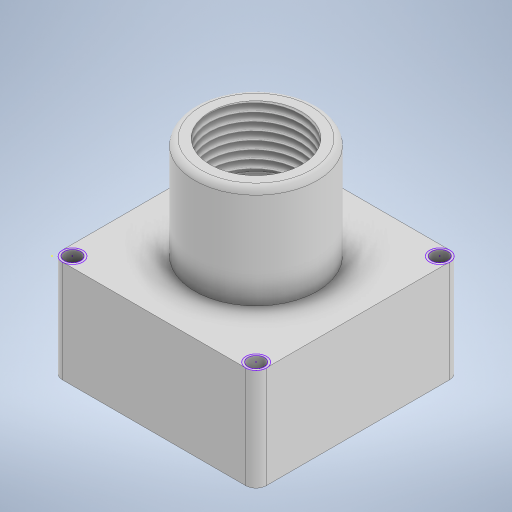
# Autodesk Inventor part: Practica1 - Jonnathan Lanuza
Saved by Autodesk Inventor 2024 (Build 280153000, 153)
## iProperties
Created: 2024-02-19
Part Number: Practica1 - Jonnathan Lanuza
Material: Generic
Document SubType Name: Modeling
Designer: Jonnathan Lanuza
Density: 1 g/cm^3
Appearance: Default
Author: Jonnathan Lanuza
Title: Practica 1 - Dinamica
Autodesk Inventor part; units mm, degrees
ref_plane "YZ Plane" through (0, 0, 0) normal (1, 0, 0) x (0, 1, 0)
ref_plane "XZ Plane" through (0, 0, 0) normal (0, 1, 0) x (-1, 0, 0)
ref_plane "XY Plane" through (0, 0, 0) normal (0, 0, 1) x (1, 0, 0)
sketch "Sketch1" plane through (0, 0, 0) normal (0, 1, 0) x (-1, 0, 0)
  point P0 (0, 0)
sketch "Sketch2" plane through (0, 0, 0) normal (0, 1, 0) x (-1, 0, 0)
  line L0 (-50, 50) -> (50, 50)
  line L1 (50, 50) -> (50, -50)
  line L2 (50, -50) -> (-50, -50)
  line L3 (-50, -50) -> (-50, 50)
  line L4 (-50, 50) -> (50, -50) construction
  line L5 (50, 50) -> (-50, -50) construction
  point P0 (0, 0)
  dimension "d0" = 100
  dimension "d1" = 100
  constraints: 12 end point, 2 midpoint, 2 parallel, 1 horizontal, 1 perpendicular
  measures "d0" distance of L1.end L2.end
  measures "d1" distance of L0.end L1.end
extrude "Extrusion1" add sketch "Sketch2" against normal blind 50
sketch "Sketch3" plane through (0, 0, 0) normal (0, 1, 0) x (1, 0, 0)
  circle A0 centre (0, 0) radius 30
  dimension "d4" = 60
  constraints: 1 centre point, 1 coincident
  measures "d4" diameter of A0
extrude "Extrusion2" add sketch "Sketch3" along normal blind 50
sketch "Sketch4" plane through (0, 50, 0) normal (0, 1, 0) x (1, 0, 0)
  point P0 (0, 0)
hole "Hole1" at (0, 50, 0) direction (0, -1, 0) diameter 45 depth 30
thread "Thread1" size "M50x4" class "6H" standard "ANSI Metric M Profile" full length
fillet "Fillet1" radius 3 1 edges at (-30, 50, 0)
sketch "Sketch9" plane through (0, 0, 0) normal (0, 1, 0) x (1, 0, 0)
  circle A0 centre (45, 45) radius 4
  circle A1 centre (45, 45) radius 5
  circle A2 centre (45, -45) radius 5
  circle A3 centre (45, -45) radius 4
  circle A4 centre (-45, 45) radius 4
  circle A5 centre (-45, 45) radius 5
  circle A6 centre (-45, -45) radius 4
  circle A7 centre (-45, -45) radius 5
  point P0 (0, 0)
  point P1 (-50, 50)
  point P2 (-50, -50)
  constraints: 8 centre point, 4 coincident
fillet "Fillet6" radius 5 1 edges at (-50, -25, 50)
fillet "Fillet7" radius 5 1 edges at (-50, -25, -50)
fillet "Fillet8" radius 5 1 edges at (50, -25, -50)
fillet "Fillet9" radius 5 1 edges at (50, -25, 50)
hole "Hole7" at (45, 0, -45) direction (0, -1, 0) diameter 8 end through all
hole "Hole8" at (45, 0, 45) direction (0, -1, 0) diameter 8 end through all
hole "Hole9" at (-45, 0, 45) direction (0, -1, 0) diameter 8 end through all
hole "Hole10" at (-45, 0, -45) direction (0, -1, 0) diameter 8 end through all
body "Solid1"
